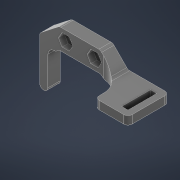
# Autodesk Inventor part: mount_battery
Saved by Autodesk Inventor 2021 (Build 250183000, 183)
## iProperties
Created: 2021-01-30
Part Number: mount_battery
Material: ABS Plastic
Document SubType Name: Modeling
Designer: User
Density: 1.06 g/cm^3
Appearance: Smooth - Black
Author: User
Autodesk Inventor part; units mm, degrees
ref_plane "YZ Plane" through (0, 0, 0) normal (1, 0, 0) x (0, 1, 0)
ref_plane "XZ Plane" through (0, 0, 0) normal (0, 1, 0) x (-1, 0, 0)
ref_plane "XY Plane" through (0, 0, 0) normal (0, 0, 1) x (1, 0, 0)
ref_plane "Work Plane1" through (0, 0, 0) normal (0, 0, 1) x (1, 0, 0)
sketch "mount_sketch" plane through (0, 0, 0) normal (0, 0, 1) x (1, 0, 0)
  circle A0 centre (42, 55.2584) radius 1.55 projected
  circle A1 centre (28, 55.2584) radius 1.55 projected
  line L0 (72.4, 52.7584) -> (52.4, 52.7584)
  line L1 (52.4, 52.7584) -> (45, 60.2584)
  line L2 (45, 60.2584) -> (25, 60.2584)
  line L3 (25, 60.2584) -> (15.4, 52.7584)
  line L4 (15.4, 52.7584) -> (15.4, 29.5584)
  line L5 (15.4, 29.5584) -> (19.4, 29.5584)
  line L6 (19.4, 29.5584) -> (19.4, 48.7584)
  line L7 (19.4, 48.7584) -> (23, 48.7584)
  line L8 (72.4, 48.7584) -> (72.4, 52.7584)
  circle A2 centre (42, -54.7416) radius 1.55 construction
  circle A3 centre (28, -54.7416) radius 1.55 construction
  line L9 (47, -54.627) -> (47, 66.2497) construction
  circle A4 centre (12, 51.2584) radius 1.55 construction
  circle A5 centre (12, -37.8416) radius 1.55 construction
  circle A6 centre (12, -54.7416) radius 1.55 construction
  circle A7 centre (29, -68.7416) radius 1.55 construction
  circle A8 centre (14, -68.7416) radius 1.55 construction
  line L10 (47, 48.7584) -> (45, 50.2584)
  line L11 (45, 50.2584) -> (25, 50.2584)
  line L12 (25, 50.2584) -> (23, 48.7584)
  line L13 (23, 48.7584) -> (47, 48.7584) construction
  line L14 (47, 48.7584) -> (72.4, 48.7584)
  point P0 (0, 0)
  dimension "d0" = 20
  dimension "d1" = 110
  dimension "d2" = 6.5
  dimension "d3" = 27.6
  dimension "d4" = 4
  dimension "d5" = 14
  dimension "d6" = 5
  dimension "d7" = 19.2
  dimension "d8" = 4
  dimension "d9" = 3.4
  dimension "d10" = 25.4
  dimension "d12" = 3
  dimension "d13" = 3
  dimension "d30" = 2
  dimension "d32" = 5
  dimension "d33" = 2
  constraints: 28 end point, 9 perpendicular, 2 horizontal, 2 vertical alignment, 1 horizontal alignment, 1 parallel, 1 point on line
  measures "d0" distance of L0.start L0.end
  measures "d1" distance of A2.centre A0.centre
  measures "d2" distance from line of A0.centre L7
  measures "d3" distance between parallel lines of L9 L6
  measures "d4" distance between parallel lines of L6 L4
  measures "d5" vertical distance of A3.centre A7.centre
  measures "d6" distance from line of L2 A0.centre
  measures "d7" distance between parallel lines of L7 L5
  measures "d8" distance of L8.start L0.start
  measures "d9" distance from line of L4 A4.centre
  measures "d10" distance between parallel lines of L8 L9
  measures "d12" horizontal distance of L1.end A0.centre
  measures "d13" horizontal distance of L2.end A1.centre
  measures "d30" horizontal distance of L2.end L7.end
  measures "d32" distance from line of L11 A0.centre
  measures "d33" horizontal distance of L1.end L10.start
extrude "mount" add sketch "mount_sketch" along normal blind 6
fillet "common" radius 2 10 edges at (15.4, 52.7584, 3) (25, 60.2584, 3) (45, 60.2584, 3) (52.4, 52.7584, 3) (15.4, 29.5584, 3) (19.4, 29.5584, 3) (23, 48.7584, 3) (25, 50.2584, 3) (45, 50.2584, 3) (47, 48.7584, 3)
fillet "battery_corner" radius 3 1 edges at (19.4, 48.7584, 3)
sketch "nuts_sketch" plane through (0, 0, 6) normal (0, 0, 1) x (1, 0, 0)
  circle A0 centre (42, 55.2584) radius 1.55 projected
  circle A1 centre (28, 55.2584) radius 1.55 projected
  line L0 (38.4782, 55.2584) -> (40.2391, 58.3084)
  line L1 (40.2391, 58.3084) -> (43.7609, 58.3084)
  line L2 (43.7609, 58.3084) -> (45.5218, 55.2584)
  line L3 (45.5218, 55.2584) -> (43.7609, 52.2084)
  line L4 (43.7609, 52.2084) -> (40.2391, 52.2084)
  line L5 (40.2391, 52.2084) -> (38.4782, 55.2584)
  line L6 (31.5218, 55.2584) -> (29.7609, 52.2084)
  line L7 (29.7609, 52.2084) -> (26.2391, 52.2084)
  line L8 (26.2391, 52.2084) -> (24.4782, 55.2584)
  line L9 (24.4782, 55.2584) -> (26.2391, 58.3084)
  line L10 (26.2391, 58.3084) -> (29.7609, 58.3084)
  line L11 (29.7609, 58.3084) -> (31.5218, 55.2584)
  point P0 (0, 0)
  dimension "d26" = 6.1
  dimension "d27" = 6.1
  constraints: 24 end point, 2 coincident, 2 horizontal alignment, 26 other
  measures "d26" distance between parallel lines of L2 L5
  measures "d27" distance between parallel lines of L8 L11
extrude "nuts" cut sketch "nuts_sketch" against normal blind 3
sketch "wall_sketch" plane through (0, 0, 6) normal (0, 0, 1) x (1, 0, 0)
  line L0 (72.4, 52.7584) -> (53.2363, 52.7584) projected
  line L1 (56.4, 52.7584) -> (56.4, 48.7584)
  line L2 (47.6667, 48.7584) -> (72.4, 48.7584) projected
  line L3 (72.4, 48.7584) -> (72.4, 52.7584) projected
  point P0 (0, 0)
  dimension "d41" = 16
  constraints: 2 end point, 2 point on line, 1 perpendicular
  measures "d41" distance between parallel lines of L1 L3
extrude "wall" add sketch "wall_sketch" along normal blind 14
fillet "wall_fillets" radius 2 3 edges at (56.4, 50.7584, 20) (72.4, 50.7584, 20) (72.4, 50.7584, 0)
sketch "fastener_slot_sketch" plane through (53.2363, 52.7584, 6) normal (0, 1, 0) x (1, 0, 0)
  line L0 (16.1637, -11) -> (13.1637, -11)
  line L1 (13.1637, -11) -> (13.1637, 3)
  line L2 (13.1637, 3) -> (16.1637, 3)
  line L3 (16.1637, 3) -> (16.1637, -11)
  line L4 (17.1637, -14) -> (5.1637, -14) projected
  line L5 (17.1637, 6) -> (0, 6) projected
  line L6 (19.1637, 4) -> (19.1637, -12) projected
  point P0 (-53.2363, 6)
  dimension "d45" = 14
  dimension "d46" = 20
  dimension "d47" = 3
  dimension "d48" = 3
  dimension "d49" = 3
  constraints: 8 end point, 2 parallel, 1 horizontal, 1 perpendicular
  measures "d45" distance of L0.end L1.end
  measures "d46" distance between parallel lines of L5 L4
  measures "d47" distance between parallel lines of L4 L0
  measures "d48" distance between parallel lines of L6 L3
  measures "d49" distance of L1.end L2.end
extrude "fastener_slot" cut sketch "fastener_slot_sketch" against normal through all
fillet "wall_support" radius 10 1 edges at (56.4, 50.7584, 6)
equation "\"d27\" = d26"
equation "\"d47\" = -0.5 * d45 + 0.5 * d46"
body "Solid1"
